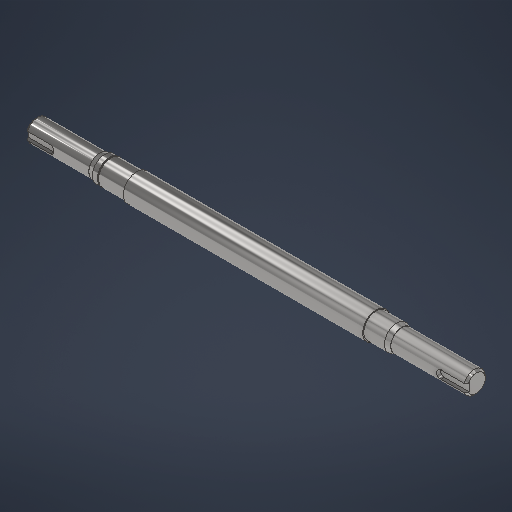
# Autodesk Inventor part: Shaft
Saved by Autodesk Inventor 2026.1 (Build 301233020, 233B)
## iProperties
Created: 2025-10-14
Part Number: Shaft
Material: Steel, High Strength, Low Alloy
Document SubType Name: Modeling
Designer: Alexander
Density: 7.85 g/cm^3
Appearance: Steel - Polished
Author: Alexander
Autodesk Inventor part; units mm, degrees
ref_plane "YZ Plane" through (0, 0, 0) normal (1, 0, 0) x (0, 1, 0)
ref_plane "XZ Plane" through (0, 0, 0) normal (0, 1, 0) x (-1, 0, 0)
sketch "Sketch1" plane through (0, 0, 0) normal (0, 0, 1) x (1, 0, 0)
  line L0 (-150.8, -12.5) -> (-140.8, -12.5)
  line L1 (-140.8, -12.5) -> (-140.8, -11.95)
  line L2 (-140.8, -11.95) -> (-139.6, -11.95)
  line L3 (-139.6, -11.95) -> (-139.6, -12.5)
  line L4 (-139.6, -12.5) -> (-113.8, -12.5)
  line L5 (-113.8, -12.5) -> (-113.8, -13.55)
  line L6 (-113.8, -13.55) -> (125.2, -13.55)
  line L7 (125.2, -13.55) -> (125.2, -12.5)
  line L8 (125.2, -12.5) -> (150.8, -12.5)
  line L9 (150.8, -12.5) -> (150.8, 0)
  line L10 (150.8, 0) -> (-150.8, 0)
  line L11 (-150.8, 0) -> (-150.8, -12.5)
  point P0 (0, 0)
  point P1 (0, 0)
  point P2 (125.2, -13.025)
  point P3 (-150.8, -6.25)
  dimension "d0" = 12.5
  dimension "d1" = 10
  dimension "d2" = 1.2
  dimension "d3" = 0.55
  dimension "d4" = 25.8
  dimension "d5" = 13.55
  dimension "d6" = 11.95
  dimension "d7" = 239
  dimension "d8" = 12.5
  dimension "d26" = 301.6
  constraints: 24 end point, 10 perpendicular, 3 midpoint, 2 coincident, 2 point on line, 1 horizontal
  measures "d0" distance of L10.end L0.start
  measures "d1" distance of L0.start L0.end
  measures "d2" distance of L1.end L2.end
  measures "d3" distance of L0.end L1.end
  measures "d4" distance of L3.end L4.end
  measures "d5" vertical distance of point (0, 0) L5.end
  measures "d6" distance from line of L10 L1.end
  measures "d7" distance of L5.end L6.end
  measures "d8" distance between parallel lines of L10 L8
  measures "d26" distance from line of point (-150.8, -6.25) L9
revolve "Revolution1" add sketch "Sketch1" angle 360 about axis through (150.8, 0, 0) along (-1, 0, 0)
sketch "Sketch2" plane through (-150.8, 0, 0) normal (-1, 0, 0) x (0, 0, 1)
  circle A0 centre (0, 0) radius 11
  point P0 (0, 0)
  dimension "d11" = 22
  constraints: 1 centre point, 1 coincident
  measures "d11" diameter of A0
extrude "Extrusion1" add sketch "Sketch2" along normal blind 64
sketch "Sketch3" plane through (150.8, 0, 0) normal (1, 0, 0) x (0, 0, -1)
  point P0 (0, 0)
sketch "Sketch4" plane through (150.8, 0, 0) normal (1, 0, 0) x (0, 0, -1)
  circle A0 centre (0, 0) radius 11
  point P0 (0, 0)
  dimension "d14" = 22
  constraints: 1 centre point, 1 coincident
  measures "d14" diameter of A0
extrude "Extrusion2" add sketch "Sketch4" along normal blind 74.4
ref_plane "Work Plane1" through (-150.8, 0, 11) normal (0, 0, 1) x (1, 0, 0)
sketch "Sketch5" plane through (-150.8, 0, 11) normal (0, 0, 1) x (1, 0, 0)
  line L0 (-64, 11) -> (-64, -11) projected
  line L1 (-64, 4) -> (-39, 4)
  line L2 (-39, 4) -> (-39, -4)
  line L3 (-39, -4) -> (-64, -4)
  line L4 (-64, -4) -> (-64, 4)
  circle A0 centre (-39, 0) radius 4
  line L5 (376, -11) -> (376, 11) projected
  line L6 (376, 4) -> (351, 4)
  line L7 (351, 4) -> (351, -4)
  line L8 (351, -4) -> (376, -4)
  line L9 (376, -4) -> (376, 4)
  circle A1 centre (351, 0) radius 4
  point P0 (150.8, 0)
  point P1 (-64, 0)
  point P2 (376, 0)
  point P3 (376, 0)
  dimension "d17" = 8
  dimension "d18" = 25
  dimension "d19" = 8
  dimension "d20" = 25
  constraints: 16 end point, 5 midpoint, 4 parallel, 2 coincident, 2 horizontal, 2 perpendicular, 2 point on line, 1 horizontal alignment, 6 other
  measures "d17" distance of L1.end L2.end
  measures "d18" distance between parallel lines of L0 L2
  measures "d19" distance of L6.end L7.end
  measures "d20" distance of L6.start L6.end
extrude "Extrusion3" cut sketch "Sketch5" against normal blind 4
chamfer "Chamfer1" distance 2 angle 45 3 edges at (-214.8, 0, -11) (225.2, -10.8101, -2.0351) (225.2, 10.8101, -2.0351)
chamfer "Chamfer2" distance 5 angle 15 1 edges at (-150.8, 12.5, 0) measured on face at (-150.3, 12.5, 0)
chamfer "Chamfer3" distance 5 angle 15 1 edges at (150.8, 12.5, 0) measured on face at (150.3, 12.5, 0)
body "Solid1"
